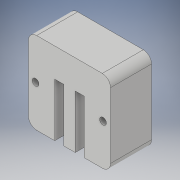
# Autodesk Inventor part: FingerProximalPhanalaxJoint
Saved by Autodesk Inventor 2018 (Build 220112000, 112)
## iProperties
Created: 2018-01-12
Part Number: FingerProximalPhanalaxJoint
Material: Generic
Document SubType Name: Modeling
Designer: iancostello
Density: 1 g/cm^3
Appearance: Default
Author: iancostello
Autodesk Inventor part; units mm, degrees
ref_plane "YZ Plane" through (0, 0, 0) normal (1, 0, 0) x (0, 1, 0)
ref_plane "XZ Plane" through (0, 0, 0) normal (0, 1, 0) x (-1, 0, 0)
ref_plane "XY Plane" through (0, 0, 0) normal (0, 0, 1) x (1, 0, 0)
sketch "Sketch2" plane through (0, 0, 0) normal (0, 1, 0) x (-1, 0, 0)
  line L0 (9.9928, 0) -> (-10.0072, 0)
  line L1 (-10.0072, 0) -> (-10.0072, -10)
  line L2 (-10.0072, -10) -> (9.9928, -10)
  line L3 (9.9928, -10) -> (9.9928, 0)
  line L4 (-0.0072, 10.1862) -> (-0.0072, -20.4961) construction
  point P0 (0, 0)
  dimension "d3" = 20
  dimension "d4" = 10
  constraints: 10 end point, 1 vertical, 1 other
  measures "d3" distance of L0.start L0.end
  measures "d4" distance of L1.end L0.end
extrude "Extrusion1" add sketch "Sketch2" along normal blind 10 and the other way blind 10
sketch "Sketch3" plane through (0, 0, 0) normal (0, 1, 0) x (-1, 0, 0)
  line L0 (-10.0072, -10) -> (9.9928, -10) projected
  circle A0 centre (-0.0072, -10) radius 6.5
  line L1 (6.4928, -10) -> (-0.0072, -10)
  line L2 (-0.0072, -3.5) -> (-0.0072, -10)
  point P0 (0, 0)
  dimension "d9" = 13
  constraints: 4 end point, 2 point on circle, 1 centre point, 1 collinear, 1 midpoint, 1 perpendicular, 1 point on line
  measures "d9" diameter of A0
revolve "Revolution1" cut sketch "Sketch3" angle 360 about axis through (0.0072, 0, -3.5) along (0, 0, -1) picked at (0.4749, -5.721) contours L2 A0 L0
sketch "Sketch4" plane through (-9.9928, 10, 0) normal (0, 0, 1) x (1, 0, 0)
  line L0 (10, -3.5) -> (10, -7) construction
  line L1 (10, -16.5) -> (10, -13) construction
  line L2 (6.5, -21.4213) -> (13.4976, -21.4213)
  line L3 (10, -7) -> (11.4, -7) construction
  line L4 (11.4, -7) -> (13.6, -7)
  line L5 (13.6, -7) -> (13.6, -20.2305)
  line L6 (13.6, -20.2305) -> (11.4, -20.2305)
  line L7 (11.4, -20.2305) -> (11.4, -7)
  line L8 (8.6, -7) -> (6.4, -7)
  line L9 (6.4, -7) -> (6.4, -20.2305)
  line L10 (6.4, -20.2305) -> (8.6, -20.2305)
  line L11 (8.6, -20.2305) -> (8.6, -7)
  point P0 (9.9928, -10)
  dimension "d11" = 3.5
  dimension "d12" = 3.5
  dimension "d20" = 1.4
  dimension "d21" = 2.2
  constraints: 24 end point, 4 symmetric about line, 2 horizontal, 2 parallel, 2 vertical, 1 coincident, 1 perpendicular
  measures "d11" distance of L0.start L0.end
  measures "d12" distance of L1.start L1.end
  measures "d20" distance of L3.start L3.end
  measures "d21" distance of L3.end L4.end
extrude "Extrusion2" cut sketch "Sketch4" against normal blind 10
sketch "Sketch5" plane through (-9.9928, 10, 0) normal (0, 0, 1) x (1, 0, 0)
  circle A0 centre (18.1773, -10) radius 0.8255
  circle A1 centre (1.7375, -10) radius 0.8255
  point P0 (9.9928, -10)
  point P1 (10, -10)
  dimension "d15" = 1.651
  dimension "d16" = 1.651
  constraints: 2 centre point
  measures "d15" diameter of A0
  measures "d16" diameter of A1
extrude "Extrusion3" cut sketch "Sketch5" against normal blind 10
fillet "Fillet1" radius 2 4 edges at (10.0072, 10, -5) (10.0072, -10, -5) (-9.9928, -10, -5) (-9.9928, 10, -5)
body "Solid1"
